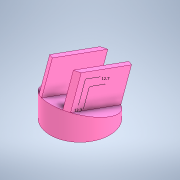
# Autodesk Inventor part: pvcBracketUpperPortionV02
Saved by Autodesk Inventor 2022.2 (Build 262287000, 287)
## iProperties
Created: 2021-10-20
Part Number: pvcBracketUpperPortionV02
Material: PC/ABS Plastic
Document SubType Name: Modeling
Designer: robst
Density: 0.357273 g/cm^3
Appearance: Pink
Author: robst
Autodesk Inventor part; units mm, degrees
ref_plane "YZ Plane" through (0, 0, 0) normal (1, 0, 0) x (0, 1, 0)
ref_plane "XZ Plane" through (0, 0, 0) normal (0, 1, 0) x (-1, 0, 0)
ref_plane "XY Plane" through (0, 0, 0) normal (0, 0, 1) x (1, 0, 0)
sketch "Sketch85" plane through (0, 0, 0) normal (0, 1, 0) x (-1, 0, 0)
  circle A0 centre (0, 0) radius 57.15
  dimension "d360" = 114.3
  constraints: 1 centre point, 1 coincident
  measures "d360" diameter of A0
extrude "Extrusion34" add sketch "Sketch85" along normal blind 60
sketch "Sketch86" plane through (0, 0, 0) normal (1, 0, 0) x (0, 1, 0)
  line L0 (0, 57.15) -> (60, 57.15) projected
  line L1 (0, -57.15) -> (0, 57.15) projected
  line L2 (60, -57.15) -> (60, 57.15) projected
  line L3 (0, -57.15) -> (60, -57.15) projected
  line L4 (51.6018, 57.15) -> (10, -57.15)
  line L5 (51.6018, 57.15) -> (51.6018, -57.15) construction
  point P0 (0, 0)
  dimension "d363" = 10
  dimension "d364" = 20
  constraints: 4 end point, 3 point on line, 1 perpendicular
  measures "d363" distance of L4.end L1.start
  measures "d364" angle of L4 L5
extrude "Extrusion35" cut sketch "Sketch86" along normal through all both and the other way through all contours L0 L2 L3 L4
sketch "Sketch90" plane through (0, 30.8009, 0) normal (0, 0.9396926, -0.3420201) x (1, 0, 0)
  ellipse E0 centre (0, 0) end of major axis (0, -60.8178) minor radius 57.15 projected
  line L0 (30.32, -51.553) -> (30.32, 51.553)
  line L1 (20.32, 56.8436) -> (20.32, -56.8436)
  arc A0 (30.32, 51.553) -> (20.32, 56.8436) centre (-1.2377, 4.0007) ccw
  arc A1 (20.32, -56.8436) -> (30.32, -51.553) centre (-1.2601, -3.9583) ccw
  point P0 (0, 10.5345)
  dimension "d378" = 10
  dimension "d379" = 20.32
  constraints: 4 end point, 4 point on circle, 2 centre point, 2 vertical, 5 other
  measures "d378" distance between parallel lines of L0 L1
  measures "d379" distance from line of L1 point (0, 0)
extrude "Extrusion38" add sketch "Sketch90" along normal blind 60 contours A1 E0 | L1 A0 L0 A1 | E0 A0
mirror "Mirror6" about plane through (0, 0, 0) normal (1, 0, 0) of "Extrusion38"
sketch "Sketch91" plane through (-30.32, 13.1687, -48.444) normal (-1, 0, 0) x (0, 0.3420201, 0.9396926)
  line L0 (0, 0) -> (0, 60) projected
  line L1 (0, 0) -> (103.106, 0) projected
  line L2 (12.7, 12.7) -> (103.106, 12.7) construction
  line L3 (12.7, 12.7) -> (12.7, 56.9582) construction
  point P0 (41.0185, -28.9434)
  dimension "d382" = 12.7
  dimension "d383" = 12.7
  constraints: 4 end point, 1 horizontal, 1 vertical
  measures "d382" distance between parallel lines of L2 L1
  measures "d383" distance from line of L2.start L0
equation "\"twoByFourWidth\" = 40.64"
equation "\"twoByFourDepth\" = 84.1375"
equation "\"azimuth\" = 55deg"
equation "\"elevationOfTwoByFour\" = 20deg"
equation "\"depthOfExtrusionForMatingToLowerHalf\" = 12.5"
equation "\"depthForWasherForMatingToCase\" = 14"
equation "\"pvcPipeInsideDiameter\" = 50.8"
equation "\"pvcPipeOutsideDiameter\" = 2.375"
equation "\"pvcPipeInsertDepth\" = 25"
equation "\"outsideDiameterOfBottom\" = 88.9"
equation "\"angleForGarage2x4\" = 20deg"
body "Solid4"
body "Solid5"
